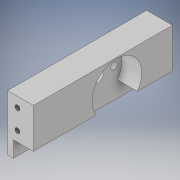
# Autodesk Inventor part: mocowanie silnika
Saved by Autodesk Inventor 2019 (Build 230136000, 136)
## iProperties
Created: 2019-09-06
Part Number: mocowanie silnika
Material: Generic
Document SubType Name: Modeling
Designer: Michal
Density: 1 g/cm^3
Appearance: Default
Author: Michal
Autodesk Inventor part; units mm, degrees
ref_plane "YZ Plane" through (0, 0, 0) normal (1, 0, 0) x (0, 1, 0)
ref_plane "XZ Plane" through (0, 0, 0) normal (0, 1, 0) x (-1, 0, 0)
ref_plane "XY Plane" through (0, 0, 0) normal (0, 0, 1) x (1, 0, 0)
sketch "Sketch1" plane through (0, 0, 0) normal (1, 0, 0) x (0, 1, 0)
  line L0 (0, 0) -> (28, 0)
  line L1 (28, 0) -> (28, -70)
  line L2 (28, -70) -> (0, -70)
  line L3 (0, -70) -> (0, 0)
  dimension "d20" = 70
  constraints: 8 end point, 2 perpendicular, 1 horizontal, 1 vertical
  measures "d20" distance of L0.end L1.end
extrude "Extrusion1" add sketch "Sketch1" along normal blind 13
sketch "Sketch2" plane through (13, 0, 0) normal (1, 0, 0) x (0, 0, -1)
  line L0 (0, 8) -> (0, 0)
  line L1 (0, 28) -> (0, 0) projected
  line L2 (0, 0) -> (70, 0) projected
  line L3 (0, 0) -> (70, 0)
  line L4 (70, 0) -> (70, 8)
  line L5 (70, 0) -> (70, 28) projected
  line L6 (0, 8) -> (70, 8)
  constraints: 8 end point, 1 collinear, 1 perpendicular, 1 point on line
extrude "Extrusion2" cut sketch "Sketch2" against normal blind 10
sketch "Sketch3" plane through (13, 0, 0) normal (1, 0, 0) x (0, 0, -1)
  line L0 (70, 0) -> (0, 0) projected
  line L1 (70, 0) -> (42, 0)
  line L2 (42, 0) -> (42, 15)
  circle A0 centre (42, 15) radius 12.5
  dimension "d21" = 28
  dimension "d22" = 15
  dimension "d23" = 25
  constraints: 4 end point, 1 centre point, 1 coincident, 1 perpendicular, 1 point on line
  measures "d21" distance of L0.start L1.end
  measures "d22" distance of L1.end L2.end
  measures "d23" diameter of A0
extrude "Extrusion3" cut sketch "Sketch3" against normal blind 10
sketch "Sketch4" plane through (3, 0, 0) normal (1, 0, 0) x (0, 0, -1)
  arc A0 (52.3562, 8) -> (31.6438, 8) centre (42, 15) ccw projected
  circle A1 centre (42, 15) radius 3.5
  line L0 (42, 15) -> (50.5, 15)
  line L1 (42, 15) -> (33.5, 15)
  circle A2 centre (33.5, 15) radius 1.7
  circle A3 centre (50.5, 15) radius 1.7
  point P0 (0, 0)
  dimension "d24" = 7
  dimension "d25" = 8.5
  dimension "d26" = 8.5
  dimension "d68" = 3.4
  dimension "d69" = 3.4
  constraints: 4 end point, 3 centre point, 2 horizontal, 1 coincident
  measures "d24" diameter of A1
  measures "d25" distance of L0.start L0.end
  measures "d26" distance of L0.start L1.end
  measures "d68" diameter of A2
  measures "d69" diameter of A3
extrude "Extrusion4" cut sketch "Sketch4" against normal blind 3
sketch "Sketch5" plane through (0, 0, -70) normal (0, 0, -1) x (-1, 0, 0)
  line L0 (0, 28) -> (-13, 28) projected
  line L1 (0, 28) -> (-5, 28)
  line L2 (-5, 28) -> (-5, 23)
  line L3 (-5, 23) -> (0, 23)
  line L4 (0, 23) -> (0, 28)
  line L5 (0, 8) -> (-5, 8)
  line L6 (-5, 8) -> (-5, 13)
  line L7 (-5, 13) -> (0, 13)
  line L8 (0, 13) -> (0, 8)
  point P0 (0, 0)
  dimension "d29" = 5
  dimension "d30" = 5
  dimension "d31" = 5
  dimension "d32" = 5
  constraints: 16 end point, 4 parallel, 2 horizontal, 2 perpendicular, 1 point on line
  measures "d29" distance of L3.end L2.end
  measures "d30" distance of L2.end L1.end
  measures "d31" distance of L6.end L7.end
  measures "d32" distance of L5.end L6.end
hole "Hole1" at (5, 13, -70) at (5, 23, -70) direction (0, 0, 1) diameter 2.4638 depth 10 tip angle 118
sketch "Sketch6" plane through (0, 0, 0) normal (0, 0, 1) x (1, 0, 0)
  line L0 (0, 28) -> (13, 28) projected
  circle A0 centre (5, 23) radius 1.2319 projected
  line L1 (0, 28) -> (5, 28)
  line L2 (5, 28) -> (5, 23)
  line L3 (5, 23) -> (0, 23)
  line L4 (0, 23) -> (0, 28)
  circle A1 centre (5, 13) radius 1.2319 projected
  line L5 (0, 8) -> (5, 8)
  line L6 (5, 8) -> (5, 13)
  line L7 (5, 13) -> (0, 13)
  line L8 (0, 13) -> (0, 8)
  point P0 (0, 0)
  point P1 (3.8741, 22.5)
  point P2 (6.1259, 22.5)
  constraints: 16 end point, 4 parallel, 2 horizontal, 2 perpendicular, 1 point on line
hole "Hole2" at (5, 23, 0) at (5, 13, 0) direction (0, 0, -1) diameter 2.4638 depth 10 tip angle 118
sketch "Sketch9" plane through (3, 8, 0) normal (0, -1, 0) x (1, 0, 0)
  line L0 (-3, 0) -> (10, 0) projected
  line L1 (10, 0) -> (5, 0)
  line L2 (5, 0) -> (5, -15)
  line L3 (5, -15) -> (10, -15)
  line L4 (10, -15) -> (10, 0)
  line L5 (10, -70) -> (10, 0) projected
  line L6 (10, -70) -> (5, -70)
  line L7 (5, -70) -> (5, -58)
  line L8 (5, -58) -> (10, -58)
  line L9 (10, -58) -> (10, -70)
  dimension "d70" = 5
  dimension "d71" = 15
  dimension "d74" = 5
  dimension "d75" = 12
  constraints: 16 end point, 4 parallel, 2 horizontal, 2 perpendicular
  measures "d70" distance of L3.end L2.end
  measures "d71" distance of L2.end L1.end
  measures "d74" distance of L7.end L8.end
  measures "d75" distance of L6.end L7.end
hole "Hole4" at (8, 8, -15) at (8, 8, -58) direction (0, 1, 0) diameter 4.1402 depth 10 tip angle 118
body "Solid1"
